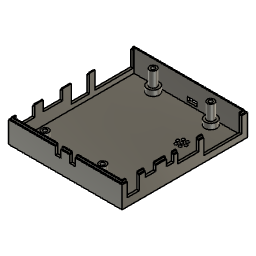
VersaTermTop (Autodesk Fusion 360 design; units mm, degrees)
Autodesk Fusion 360 part; units mm, degrees
box "BoxPrimitive1" add length 104.5 width 94.5 height 20.6 placed x (0, 1, 0) y (-1, 0, 0) z (0, 0, 1) at (94.5, 0, 0) makes body 1
shell "Shell1" thickness 2 removed faces 1 at (31.5, 34.8333, 20.6) on bodies 1
sketch "Sketch3" plane through (0, 0, 2) normal (0, 0, 1) x (-1, 0, 0)
  line L0 (-92.5, -102.5) -> (-2, -102.5)
  line L1 (-2, -102.5) -> (-2, -2)
  line L2 (-2, -2) -> (-92.5, -2)
  line L3 (-92.5, -2) -> (-92.5, -102.5)
  circle A0 centre (-23.25, -97.25) radius 5
  dimension "d7" = 10
  dimension "d8" = 5.25
  dimension "d9" = 21.25
  measures "d7" diameter of A0
  measures "d8" distance of L0 A0.centre
  measures "d9" distance of L1 A0.centre
extrude "Extrude1" add sketch "Sketch3" along normal blind 4.6 contours A0 bodies 1
sketch "Sketch16" plane through (0, 0, 6.6) normal (0, 0, 1) x (-1, 0, 0)
  circle A0 centre (-23.25, -97.25) radius 5
  circle A1 centre (-23.25, -97.25) radius 3
  dimension "d42" = 6
  constraint concentric A0 A1
  measures "d42" diameter of A1
extrude "Extrude7" add sketch "Sketch16" along normal blind 12.4 contours A1 bodies 1
sketch "Sketch18" plane through (0, 0, 2) normal (0, 0, 1) x (-1, 0, 0)
  circle A0 centre (-23.25, -97.25) radius 5
  line L0 (-92.5, -102.5) -> (-2, -102.5)
  line L1 (-2, -102.5) -> (-2, -2)
  line L2 (-2, -2) -> (-92.5, -2)
  line L3 (-92.5, -2) -> (-92.5, -102.5)
  circle A1 centre (-23.25, -97.25) radius 3.125
  dimension "d49" = 6.25
  constraint concentric A0 A1
  measures "d49" diameter of A1
extrude "Extrude8" cut sketch "Sketch18" against normal blind 3.1 from surface at 1.1 contours A1 bodies 1
sketch "Sketch20" plane through (0, 0, 3.1) normal (0, 0, -1) x (1, 0, 0)
  circle A0 centre (23.25, -97.25) radius 3.125
  circle A1 centre (23.25, -97.25) radius 1.55
  dimension "d56" = 3.1
  constraint concentric A0 A1
  measures "d56" diameter of A1
extrude "Extrude10" cut sketch "Sketch20" against normal blind 17 contours A1 bodies 1
pattern_linear "R-Pattern3" count 2 spacing 90 along (0, -1, 0) count 2 spacing 48 along (1, 0, 0) of "Extrude1", "Extrude7", "Extrude8", "Extrude10"
chamfer "Chamfer2" distance 1 angle 45 4 edges at (94.5, 52.25, 0) (47.25, 0, 0) (47.25, 104.5, 0) (0, 52.25, 0) on bodies 1
sketch "Sketch39" plane through (0, 0, 20.6) normal (0, 0, 1) x (-1, 0, 0)
  line L0 (-92.5, -102.5) -> (-92.5, -2)
  line L1 (-92.5, -2) -> (-2, -2)
  line L2 (-2, -2) -> (-2, -102.5)
  line L3 (-2, -102.5) -> (-92.5, -102.5)
  line L4 (-94.5, -104.5) -> (0, -104.5)
  line L5 (0, -104.5) -> (0, 0)
  line L6 (0, 0) -> (-94.5, 0)
  line L7 (-94.5, 0) -> (-94.5, -104.5)
  line L8 (0, -104.5) -> (-94.5, -104.5)
  line L9 (-94.5, -104.5) -> (-94.5, 0)
  line L10 (-94.5, 0) -> (0, 0)
  line L11 (0, 0) -> (0, -104.5)
  line L12 (-93.4, -1.1) -> (-1.1, -1.1)
  line L13 (-1.1, -1.1) -> (-1.1, -103.4)
  line L14 (-1.1, -103.4) -> (-93.4, -103.4)
  line L15 (-93.4, -103.4) -> (-93.4, -1.1)
  dimension "d89" = 1.1
  constraint horizontal L8
  constraint vertical L9
  constraint horizontal L10
  constraint vertical L11
  constraint coincident L6.end L7.start
  constraint coincident L4.end L5.start
extrude "Extrude15" cut sketch "Sketch39" against normal blind 1.6 contours L4 L5 L6 L7 L8 L9 L10 L11 bodies 1
sketch "Sketch27" plane through (94.5, 0, 0) normal (1, 0, 0) x (0, 1, 0)
  line L0 (104.5, 1) -> (104.5, 19)
  line L1 (0, 19) -> (0, 1)
  line L2 (4.39, 20.6) -> (14.39, 20.6)
  line L3 (14.39, 20.6) -> (14.39, 7.6)
  line L4 (14.39, 7.6) -> (4.39, 7.6)
  line L5 (4.39, 7.6) -> (4.39, 20.6)
  line L6 (0, 1) -> (104.5, 1)
  line L7 (104.5, 19) -> (0, 19)
  line L8 (1.1, 20.6) -> (103.4, 20.6)
  dimension "d69" = 13
  dimension "d70" = 10
  dimension "d79" = 4.39
  constraint horizontal L2
  constraint vertical L3
  constraint horizontal L4
  constraint vertical L5
  constraint collinear L2 L8
  measures "d69" distance of L2 L4
  measures "d70" distance of L3 L5
  measures "d79" distance of L1 L5
extrude "Extrude12" cut sketch "Sketch27" against normal blind 2 contours L2 L3 L5 L7 L8 | L3 L4 L5 L7 bodies 1
sketch "Sketch28" plane through (94.5, 0, 0) normal (1, 0, 0) x (0, 1, 0)
  line L0 (0, 19) -> (0, 1)
  line L1 (104.5, 1) -> (104.5, 19)
  line L2 (19.465, 20.6) -> (28.165, 20.6)
  line L3 (28.165, 20.6) -> (28.165, 14.7)
  line L4 (28.165, 14.7) -> (19.465, 14.7)
  line L5 (19.465, 14.7) -> (19.465, 20.6)
  line L6 (4.39, 7.6) -> (4.39, 19)
  line L7 (14.39, 19) -> (14.39, 7.6)
  line L8 (14.39, 7.6) -> (4.39, 7.6)
  line L9 (0, 1) -> (104.5, 1)
  line L10 (4.39, 19) -> (0, 19)
  line L11 (104.5, 19) -> (14.39, 19)
  line L12 (14.39, 20.6) -> (103.4, 20.6)
  dimension "d75" = 8.7
  dimension "d76" = 5.9
  dimension "d80" = 19.465
  constraint horizontal L2
  constraint vertical L3
  constraint horizontal L4
  constraint vertical L5
  constraint collinear L2 L12
  measures "d75" distance of L3 L5
  measures "d76" distance of L2 L4
  measures "d80" distance of L0 L5
extrude "Extrude13" cut sketch "Sketch28" against normal blind 2 contours L2 L3 L5 L11 L12 | L3 L4 L5 L11 bodies 1
sketch "Sketch41" plane through (0, 0, 0) normal (-1, 0, 0) x (0, -1, 0)
  line L0 (-104.5, 19) -> (-104.5, 1)
  line L1 (0, 1) -> (0, 19)
  line L2 (-65.35, 20.6) -> (-50.35, 20.6)
  line L3 (-50.35, 20.6) -> (-50.35, 5.8)
  line L4 (-50.35, 5.8) -> (-65.35, 5.8)
  line L5 (-65.35, 5.8) -> (-65.35, 20.6)
  line L6 (-104.5, 1) -> (0, 1)
  line L7 (0, 19) -> (-104.5, 19)
  line L8 (-28.165, 20.6) -> (-103.4, 20.6)
  dimension "d97" = 14.8
  dimension "d98" = 15
  dimension "d102" = 39.15
  constraint horizontal L2
  constraint vertical L3
  constraint horizontal L4
  constraint vertical L5
  constraint collinear L2 L8
  measures "d97" distance of L2 L4
  measures "d98" distance of L3 L5
  measures "d102" distance of L0 L5
extrude "Extrude17" cut sketch "Sketch41" against normal blind 2 contours L3 L4 L5 L7 | L2 L3 L5 L7 L8 bodies 1
sketch "Sketch42" plane through (0, 0, 0) normal (-1, 0, 0) x (0, -1, 0)
  line L0 (-65.35, 5.8) -> (-65.35, 19)
  line L1 (-104.5, 19) -> (-104.5, 1)
  line L2 (0, 1) -> (0, 19)
  line L3 (-50.35, 19) -> (-50.35, 5.8)
  line L4 (-50.35, 5.8) -> (-65.35, 5.8)
  line L5 (-42.94, 20.6) -> (-26.94, 20.6)
  line L6 (-26.94, 20.6) -> (-26.94, 12)
  line L7 (-26.94, 12) -> (-42.94, 12)
  line L8 (-42.94, 12) -> (-42.94, 20.6)
  line L9 (-104.5, 1) -> (0, 1)
  line L10 (-65.35, 19) -> (-104.5, 19)
  line L11 (0, 19) -> (-50.35, 19)
  line L12 (-28.165, 20.6) -> (-103.4, 20.6)
  dimension "d103" = 16
  dimension "d104" = 8.6
  dimension "d105" = 26.94
  constraint horizontal L5
  constraint vertical L6
  constraint horizontal L7
  constraint vertical L8
  constraint collinear L5 L12
  measures "d103" distance of L6 L8
  measures "d104" distance of L5 L7
  measures "d105" distance of L2 L6
extrude "Extrude18" cut sketch "Sketch42" against normal blind 2 contours L6 L7 L8 L11 | L5 L6 L8 L11 L12 bodies 1
sketch "Sketch43" plane through (0, 0, 0) normal (-1, 0, 0) x (0, -1, 0)
  line L0 (-42.94, 12) -> (-42.94, 19)
  line L1 (-50.35, 19) -> (-50.35, 5.8)
  line L2 (-50.35, 5.8) -> (-65.35, 5.8)
  line L3 (-65.35, 5.8) -> (-65.35, 19)
  line L4 (-104.5, 19) -> (-104.5, 1)
  line L5 (0, 1) -> (0, 19)
  line L6 (-26.94, 19) -> (-26.94, 12)
  line L7 (-26.94, 12) -> (-42.94, 12)
  line L8 (-19.83, 20.6) -> (-4.33, 20.6)
  line L9 (-4.33, 20.6) -> (-4.33, 11.5)
  line L10 (-4.33, 11.5) -> (-19.83, 11.5)
  line L11 (-19.83, 11.5) -> (-19.83, 20.6)
  line L12 (-104.5, 1) -> (0, 1)
  line L13 (-42.94, 19) -> (-50.35, 19)
  line L14 (-65.35, 19) -> (-104.5, 19)
  line L15 (0, 19) -> (-26.94, 19)
  line L16 (-2, 20.6) -> (-26.94, 20.6)
  dimension "d108" = 4.33
  dimension "d109" = 15.5
  dimension "d110" = 9.1
  constraint horizontal L8
  constraint vertical L9
  constraint horizontal L10
  constraint vertical L11
  constraint collinear L8 L16
  measures "d108" distance of L5 L9
  measures "d109" distance of L9 L11
  measures "d110" distance of L8 L10
extrude "Extrude19" cut sketch "Sketch43" against normal blind 2 contours L9 L10 L11 L15 | L8 L9 L11 L15 L16 bodies 1
sketch "Sketch44" plane through (0, 0, 0) normal (-1, 0, 0) x (0, -1, 0)
  line L0 (-19.83, 11.5) -> (-19.83, 19)
  line L1 (-26.94, 19) -> (-26.94, 12)
  line L2 (-26.94, 12) -> (-42.94, 12)
  line L3 (-42.94, 12) -> (-42.94, 19)
  line L4 (-50.35, 19) -> (-50.35, 5.8)
  line L5 (-50.35, 5.8) -> (-65.35, 5.8)
  line L6 (-65.35, 5.8) -> (-65.35, 19)
  line L7 (-104.5, 19) -> (-104.5, 1)
  line L8 (0, 1) -> (0, 19)
  line L9 (-4.33, 19) -> (-4.33, 11.5)
  line L10 (-4.33, 11.5) -> (-19.83, 11.5)
  line L11 (-101.776, 20.6) -> (-69.966, 20.6)
  line L12 (-69.966, 20.6) -> (-69.966, 6.05)
  line L13 (-69.966, 6.05) -> (-101.776, 6.05)
  line L14 (-101.776, 6.05) -> (-101.776, 20.6)
  line L15 (-104.5, 1) -> (0, 1)
  line L16 (-19.83, 19) -> (-26.94, 19)
  line L17 (-42.94, 19) -> (-50.35, 19)
  line L18 (-65.35, 19) -> (-104.5, 19)
  line L19 (0, 19) -> (-4.33, 19)
  line L20 (-28.165, 20.6) -> (-103.4, 20.6)
  dimension "d113" = 31.81
  dimension "d114" = 14.55
  dimension "d115" = 2.724
  constraint horizontal L11
  constraint vertical L12
  constraint horizontal L13
  constraint vertical L14
  constraint collinear L11 L20
  measures "d113" distance of L12 L14
  measures "d114" distance of L11 L13
  measures "d115" distance of L7 L14
extrude "Extrude20" cut sketch "Sketch44" against normal blind 2 contours L12 L13 L14 L18 | L11 L12 L14 L18 L20 bodies 1
sketch "Sketch45" plane through (94.5, 0, 0) normal (1, 0, 0) x (0, 1, 0)
  line L0 (46.5, 20.6) -> (64, 20.6)
  line L1 (64, 20.6) -> (64, 10.9)
  line L2 (64, 10.9) -> (46.5, 10.9)
  line L3 (46.5, 10.9) -> (46.5, 20.6)
  line L4 (104.5, 1) -> (104.5, 18.5)
  line L5 (19.465, 14.7) -> (19.465, 19)
  line L6 (14.39, 19) -> (14.39, 7.6)
  line L7 (14.39, 7.6) -> (4.39, 7.6)
  line L8 (4.39, 7.6) -> (4.39, 19)
  line L9 (0, 19) -> (0, 1)
  line L10 (0, 1) -> (104.5, 1)
  line L11 (104.5, 1) -> (104.5, 19)
  line L12 (28.165, 19) -> (28.165, 14.7)
  line L13 (28.165, 14.7) -> (19.465, 14.7)
  line L14 (19.465, 19) -> (14.39, 19)
  line L15 (4.39, 19) -> (0, 19)
  line L16 (104.5, 19) -> (28.165, 19)
  line L17 (28.165, 20.6) -> (103.4, 20.6)
  dimension "d118" = 40.5
  dimension "d119" = 17.5
  dimension "d120" = 9.7
  constraint horizontal L0
  constraint vertical L1
  constraint horizontal L2
  constraint vertical L3
  constraint collinear L0 L17
  measures "d118" distance of L1 L4
  measures "d119" distance of L1 L3
  measures "d120" distance of L0 L2
extrude "Extrude21" cut sketch "Sketch45" against normal blind 2 contours L0 L1 L3 L16 L17 | L1 L2 L3 L16 bodies 1
sketch "Sketch46" plane through (94.5, 0, 0) normal (1, 0, 0) x (0, 1, 0)
  line L0 (46.5, 10.9) -> (46.5, 19)
  line L1 (28.165, 19) -> (28.165, 14.7)
  line L2 (28.165, 14.7) -> (19.465, 14.7)
  line L3 (19.465, 14.7) -> (19.465, 19)
  line L4 (14.39, 19) -> (14.39, 7.6)
  line L5 (14.39, 7.6) -> (4.39, 7.6)
  line L6 (4.39, 7.6) -> (4.39, 19)
  line L7 (0, 19) -> (0, 1)
  line L8 (0, 1) -> (104.5, 1)
  line L9 (104.5, 1) -> (104.5, 19)
  line L10 (64, 19) -> (64, 10.9)
  line L11 (64, 10.9) -> (46.5, 10.9)
  line L12 (68.186, 20.6) -> (99.746, 20.6)
  line L13 (99.746, 20.6) -> (99.746, 6.05)
  line L14 (99.746, 6.05) -> (68.186, 6.05)
  line L15 (68.186, 6.05) -> (68.186, 20.6)
  line L16 (46.5, 19) -> (28.165, 19)
  line L17 (19.465, 19) -> (14.39, 19)
  line L18 (4.39, 19) -> (0, 19)
  line L19 (104.5, 19) -> (64, 19)
  line L20 (64, 20.6) -> (103.4, 20.6)
  dimension "d124" = 4.754
  dimension "d125" = 31.56
  dimension "d126" = 14.55
  constraint horizontal L12
  constraint vertical L13
  constraint horizontal L14
  constraint vertical L15
  constraint collinear L12 L20
  measures "d124" distance of L9 L13
  measures "d125" distance of L13 L15
  measures "d126" distance of L12 L14
extrude "Extrude22" cut sketch "Sketch46" against normal blind 2 contours L13 L14 L15 L19 | L12 L13 L15 L19 L20 bodies 1
sketch "Sketch47" plane through (94.5, 0, 0) normal (1, 0, 0) x (0, 1, 0)
  line L0 (68.186, 6.05) -> (68.186, 19)
  line L1 (64, 19) -> (64, 10.9)
  line L2 (64, 10.9) -> (46.5, 10.9)
  line L3 (46.5, 10.9) -> (46.5, 19)
  line L4 (28.165, 19) -> (28.165, 14.7)
  line L5 (28.165, 14.7) -> (19.465, 14.7)
  line L6 (19.465, 14.7) -> (19.465, 19)
  line L7 (14.39, 19) -> (14.39, 7.6)
  line L8 (14.39, 7.6) -> (4.39, 7.6)
  line L9 (4.39, 7.6) -> (4.39, 19)
  line L10 (0, 19) -> (0, 1)
  line L11 (0, 1) -> (104.5, 1)
  line L12 (104.5, 1) -> (104.5, 19)
  line L13 (99.746, 19) -> (99.746, 6.05)
  line L14 (99.746, 6.05) -> (68.186, 6.05)
  line L15 (37.12, 20.6) -> (43.12, 20.6)
  line L16 (43.12, 20.6) -> (43.12, 13.6)
  line L17 (43.12, 13.6) -> (37.12, 13.6)
  line L18 (37.12, 13.6) -> (37.12, 20.6)
  line L19 (68.186, 19) -> (64, 19)
  line L20 (46.5, 19) -> (28.165, 19)
  line L21 (19.465, 19) -> (14.39, 19)
  line L22 (4.39, 19) -> (0, 19)
  line L23 (104.5, 19) -> (99.746, 19)
  line L24 (28.165, 20.6) -> (46.5, 20.6)
  dimension "d129" = 6
  dimension "d130" = 7
  dimension "d131" = 37.12
  constraint horizontal L15
  constraint vertical L16
  constraint horizontal L17
  constraint vertical L18
  constraint collinear L15 L24
  measures "d129" distance of L16 L18
  measures "d130" distance of L15 L17
  measures "d131" distance of L10 L18
extrude "Extrude23" cut sketch "Sketch47" against normal blind 2 contours L15 L16 L18 L20 L24 | L16 L17 L18 L20 bodies 1
sketch "Sketch48" plane through (0, 0, 2) normal (0, 0, 1) x (-1, 0, 0)
  circle A0 centre (-71.25, -7.25) radius 5
  circle A1 centre (-71.25, -97.25) radius 5
  circle A2 centre (-23.25, -7.25) radius 5
  circle A3 centre (-23.25, -97.25) radius 5
  line L0 (-92.5, -102.5) -> (-2, -102.5)
  line L1 (-2, -102.5) -> (-2, -2)
  line L2 (-2, -2) -> (-92.5, -2)
  line L3 (-92.5, -2) -> (-92.5, -102.5)
  circle A4 centre (-73.37, -14.47) radius 3.5
  dimension "d134" = 19.13
  dimension "d135" = 7
  dimension "d136" = 12.47
  measures "d134" distance of L3 A4.centre
  measures "d135" diameter of A4
  measures "d136" distance of L2 A4.centre
sketch "Sketch49" plane through (0, 0, 0) normal (0, -1, 0) x (1, 0, 0)
  line L0 (0, 1) -> (94.5, 1)
  line L1 (94.5, 1) -> (94.5, 19)
  line L2 (0, 19) -> (0, 1)
  line L3 (51, 20.6) -> (55.5, 20.6)
  line L4 (55.5, 20.6) -> (55.5, 12.8)
  line L5 (55.5, 12.8) -> (51, 12.8)
  line L6 (51, 12.8) -> (51, 20.6)
  line L7 (94.5, 19) -> (0, 19)
  line L8 (1.1, 20.6) -> (93.4, 20.6)
  dimension "d137" = 39
  dimension "d138" = 4.5
  dimension "d139" = 7.8
  constraint horizontal L3
  constraint vertical L4
  constraint horizontal L5
  constraint vertical L6
  constraint collinear L3 L8
  measures "d137" distance of L1 L4
  measures "d138" distance of L4 L6
  measures "d139" distance of L3 L5
extrude "Extrude24" cut sketch "Sketch49" against normal blind 2 contours L4 L5 L6 L7 | L3 L4 L6 L7 L8 bodies 1
sketch "Sketch50" plane through (0, 0, 0) normal (0, -1, 0) x (1, 0, 0)
  line L0 (51, 12.8) -> (51, 19)
  line L1 (0, 19) -> (0, 1)
  line L2 (0, 1) -> (94.5, 1)
  line L3 (94.5, 1) -> (94.5, 19)
  line L4 (55.5, 19) -> (55.5, 12.8)
  line L5 (55.5, 12.8) -> (51, 12.8)
  line L6 (39, 20.6) -> (43.5, 20.6)
  line L7 (43.5, 20.6) -> (43.5, 12.8)
  line L8 (43.5, 12.8) -> (39, 12.8)
  line L9 (39, 12.8) -> (39, 20.6)
  line L10 (51, 19) -> (0, 19)
  line L11 (94.5, 19) -> (55.5, 19)
  line L12 (1.1, 20.6) -> (51, 20.6)
  dimension "d142" = 51
  dimension "d143" = 4.5
  dimension "d144" = 7.8
  constraint horizontal L6
  constraint vertical L7
  constraint horizontal L8
  constraint vertical L9
  constraint collinear L6 L12
  measures "d142" distance of L3 L7
  measures "d143" distance of L7 L9
  measures "d144" distance of L6 L8
extrude "Extrude25" cut sketch "Sketch50" against normal blind 2 contours L6 L7 L9 L10 L12 | L7 L8 L9 L10 bodies 1
extrude "Extrude26" add sketch "Sketch48" along normal blind 6 separate body contours A0 A4 | A0 A4 picked at (-72.1915, -11.8436) picked at (-71.939, -13.8039) makes body 2
combine "Combine1" operation cut target body 1 tool bodies 2
sketch "Sketch57" plane through (0, 0, 2) normal (0, 0, 1) x (-1, 0, 0)
  arc A0 (-70.6903, -12.2186) -> (-74.4071, -11.1272) centre (-71.25, -7.25) ccw
  arc A1 (-70.6903, -12.2186) -> (-74.4071, -11.1272) centre (-73.37, -14.47) ccw
  circle A2 centre (-71.25, -97.25) radius 5
  circle A3 centre (-23.25, -7.25) radius 5
  circle A4 centre (-23.25, -97.25) radius 5
  line L0 (-92.5, -102.5) -> (-2, -102.5)
  line L1 (-2, -102.5) -> (-2, -2)
  line L2 (-2, -2) -> (-92.5, -2)
  line L3 (-92.5, -2) -> (-92.5, -102.5)
  circle A5 centre (-72.05, -72.25) radius 1.25
  dimension "d149" = 2.5
  dimension "d150" = 30.25
  dimension "d151" = 20.45
  measures "d149" diameter of A5
  measures "d150" distance of L0 A5.centre
  measures "d151" distance of L3 A5.centre
extrude "Extrude27" cut sketch "Sketch57" against normal blind 2 contours A5 bodies 1
sketch "Sketch58" plane through (0, 0, 2) normal (0, 0, 1) x (-1, 0, 0)
  circle A0 centre (-72.05, -72.25) radius 1.25
  arc A1 (-70.6903, -12.2186) -> (-74.4071, -11.1272) centre (-71.25, -7.25) ccw
  arc A2 (-70.6903, -12.2186) -> (-74.4071, -11.1272) centre (-73.37, -14.47) ccw
  circle A3 centre (-71.25, -97.25) radius 5
  circle A4 centre (-23.25, -7.25) radius 5
  circle A5 centre (-23.25, -97.25) radius 5
  line L0 (-92.5, -102.5) -> (-2, -102.5)
  line L1 (-2, -102.5) -> (-2, -2)
  line L2 (-2, -2) -> (-92.5, -2)
  line L3 (-92.5, -2) -> (-92.5, -102.5)
  circle A6 centre (-68.55, -72.25) radius 1.25
  dimension "d154" = 23.95
  dimension "d155" = 30.25
  dimension "d158" = 2.5
  measures "d154" distance of L3 A6.centre
  measures "d155" distance of L0 A6.centre
  measures "d158" diameter of A6
extrude "Extrude28" cut sketch "Sketch58" against normal blind 2 contours A6 bodies 1
pattern_circular "C-Pattern1" count 6 over 360 about axis through (72.05, 72.25, 2) along (0, 0, -1) of 1 faces at (68.1519, 71.0651, 0.6667) on bodies 1
sketch "Sketch61" plane through (0, 0, 2) normal (0, 0, 1) x (1, 0, 0)
  circle A0 centre (72.05, 65.25) radius 1.25
  line L0 (92.5, 68.186) -> (92.5, 100.246)
  line L1 (2, 102.5) -> (92.5, 102.5)
  dimension "d163" = 20.45
  dimension "d164" = 2.5
  dimension "d165" = 37.25
  measures "d163" distance of A0.centre L0
  measures "d164" diameter of A0
  measures "d165" distance of A0.centre L1
extrude "Extrude29" [suppressed]
pattern_circular "C-Pattern2" [suppressed]
sketch "Sketch62" plane through (0, 104.5, 0) normal (0, 1, 0) x (-1, 0, 0)
  line L0 (0, 19) -> (-94.5, 19)
  line L1 (-94.5, 19) -> (-94.5, 1)
  line L2 (-94.5, 1) -> (0, 1)
  line L3 (0, 1) -> (0, 19)
  line L4 (-54.5, 7.5) -> (-46.5, 7.5)
  line L5 (-46.5, 7.5) -> (-46.5, 4)
  line L6 (-46.5, 4) -> (-54.5, 4)
  line L7 (-54.5, 4) -> (-54.5, 7.5)
  dimension "d171" = 11.5
  dimension "d172" = 8
  dimension "d173" = 3.5
  dimension "d206" = 40
  constraint horizontal L4
  constraint vertical L5
  constraint horizontal L6
  constraint vertical L7
  measures "d171" distance of L0 L4
  measures "d172" distance of L5 L7
  measures "d173" distance of L4 L6
  measures "d206" distance of L1 L4.start
extrude "Extrude30" cut sketch "Sketch62" against normal blind 2 contours L4 L5 L6 L7 bodies 1
sketch "Sketch63" plane through (94.5, 0, 0) normal (1, 0, 0) x (0, 1, 0)
  line L0 (43.12, 19) -> (43.12, 13.6)
  line L1 (43.12, 13.6) -> (37.12, 13.6)
  line L2 (37.12, 13.6) -> (37.12, 19)
  line L3 (37.12, 19) -> (28.165, 19)
  line L4 (28.165, 19) -> (28.165, 14.7)
  line L5 (28.165, 14.7) -> (19.465, 14.7)
  line L6 (19.465, 14.7) -> (19.465, 19)
  line L7 (19.465, 19) -> (14.39, 19)
  line L8 (14.39, 19) -> (14.39, 7.6)
  line L9 (14.39, 7.6) -> (4.39, 7.6)
  line L10 (4.39, 7.6) -> (4.39, 19)
  line L11 (4.39, 19) -> (0, 19)
  line L12 (0, 19) -> (0, 1)
  line L13 (0, 1) -> (104.5, 1)
  line L14 (104.5, 1) -> (104.5, 19)
  line L15 (104.5, 19) -> (99.746, 19)
  line L16 (99.746, 19) -> (99.746, 6.05)
  line L17 (99.746, 6.05) -> (68.186, 6.05)
  line L18 (68.186, 6.05) -> (68.186, 19)
  line L19 (68.186, 19) -> (64, 19)
  line L20 (64, 19) -> (64, 10.9)
  line L21 (64, 10.9) -> (46.5, 10.9)
  line L22 (46.5, 10.9) -> (46.5, 19)
  line L23 (46.5, 19) -> (43.12, 19)
  line L24 (68.186, 6.05) -> (99.746, 6.05)
  line L25 (99.746, 6.05) -> (99.746, 1)
  line L26 (99.746, 1) -> (68.186, 1)
  line L27 (68.186, 1) -> (68.186, 6.05)
  constraint horizontal L24
  constraint vertical L25
  constraint horizontal L26
  constraint vertical L27
  constraint coincident L13 L25.end
  constraint coincident L17.end L18.start
  constraint collinear L16 L25
extrude "Extrude31" [suppressed]
draft "Draft1" [suppressed]
sketch "Sketch70" plane through (94.5, 0, 0) normal (1, 0, 0) x (0, 1, 0)
  line L0 (68.186, 6.05) -> (68.186, 19)
  line L1 (68.186, 19) -> (64, 19)
  line L2 (64, 19) -> (64, 10.9)
  line L3 (64, 10.9) -> (46.5, 10.9)
  line L4 (46.5, 10.9) -> (46.5, 19)
  line L5 (46.5, 19) -> (43.12, 19)
  line L6 (43.12, 19) -> (43.12, 13.6)
  line L7 (43.12, 13.6) -> (37.12, 13.6)
  line L8 (37.12, 13.6) -> (37.12, 19)
  line L9 (37.12, 19) -> (28.165, 19)
  line L10 (28.165, 19) -> (28.165, 14.7)
  line L11 (28.165, 14.7) -> (19.465, 14.7)
  line L12 (19.465, 14.7) -> (19.465, 19)
  line L13 (19.465, 19) -> (14.39, 19)
  line L14 (14.39, 19) -> (14.39, 7.6)
  line L15 (14.39, 7.6) -> (4.39, 7.6)
  line L16 (4.39, 7.6) -> (4.39, 19)
  line L17 (4.39, 19) -> (0, 19)
  line L18 (0, 19) -> (0, 1)
  line L19 (0, 1) -> (104.5, 1)
  line L20 (104.5, 1) -> (104.5, 19)
  line L21 (104.5, 19) -> (99.746, 19)
  line L22 (99.746, 19) -> (99.746, 6.05)
  line L23 (99.746, 19) -> (104.5, 19)
  line L24 (104.5, 19) -> (104.5, 6.05)
  line L25 (104.5, 6.05) -> (99.746, 6.05)
  line L26 (99.746, 6.05) -> (99.746, 19)
  line L27 (68.186, 1.0007) -> (68.186, 6.05)
  line L28 (99.746, 6.05) -> (99.746, 1.0007)
  line L29 (99.746, 1.0007) -> (68.186, 1.0007)
  constraint horizontal L23
  constraint vertical L24
  constraint vertical L26
  constraint coincident L20 L24.end
  constraint coincident L21.end L22.start
extrude "Extrude35" [suppressed]
draft "Draft2" [suppressed]
loft "Loft2" [suppressed]
sketch "Sketch69" plane through (94.5, 0, 0) normal (1, 0, 0) x (0, 1, 0)
  line L0 (68.186, 1.0007) -> (68.186, 6.05)
  line L1 (68.186, 6.05) -> (68.186, 19)
  line L2 (68.186, 19) -> (64, 19)
  line L3 (64, 19) -> (64, 10.9)
  line L4 (64, 10.9) -> (46.5, 10.9)
  line L5 (46.5, 10.9) -> (46.5, 19)
  line L6 (46.5, 19) -> (43.12, 19)
  line L7 (43.12, 19) -> (43.12, 13.6)
  line L8 (43.12, 13.6) -> (37.12, 13.6)
  line L9 (37.12, 13.6) -> (37.12, 19)
  line L10 (37.12, 19) -> (28.165, 19)
  line L11 (28.165, 19) -> (28.165, 14.7)
  line L12 (28.165, 14.7) -> (19.465, 14.7)
  line L13 (19.465, 14.7) -> (19.465, 19)
  line L14 (19.465, 19) -> (14.39, 19)
  line L15 (14.39, 19) -> (14.39, 7.6)
  line L16 (14.39, 7.6) -> (4.39, 7.6)
  line L17 (4.39, 7.6) -> (4.39, 19)
  line L18 (4.39, 19) -> (0, 19)
  line L19 (0, 19) -> (0, 1)
  line L20 (0, 1) -> (104.5, 1)
  line L21 (64, 19) -> (68.186, 19)
  line L22 (68.186, 19) -> (68.186, 6.05)
  line L23 (68.186, 6.05) -> (64, 6.05)
  line L24 (64, 6.05) -> (64, 19)
  line L25 (104.5, 1) -> (104.5, 19)
  line L26 (99.746, 1.0007) -> (68.186, 1.0007)
  line L27 (104.473, 6.05) -> (99.746, 1.0007)
  line L28 (104.5, 19) -> (104.473, 19)
  line L29 (104.473, 19) -> (104.473, 6.05)
  constraint horizontal L21
  constraint vertical L22
  constraint horizontal L23
  constraint vertical L24
  constraint coincident L0.end L1.start
  constraint coincident L2.end L3.start
extrude "Extrude38" [suppressed]
draft "Draft6" [suppressed]
loft "Loft4" [suppressed]
loft "Loft3" [suppressed]
